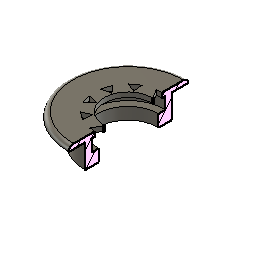
capuchon (Autodesk Fusion 360 design; units mm, degrees)
Autodesk Fusion 360 part; units mm, degrees
sketch "Esquisse1" plane through (0, 0, 0) normal (0, 1, 0) x (1, 0, 0)
  circle A0 centre (0, 0) radius 18.15
  circle A1 centre (0, 0) radius 15.5
  dimension "d1" = 36.3
  dimension "d2" = 31
  constraint coincident A0.centre A1.centre
  constraint concentric A0 A1
  measures "d1" diameter of A0
  measures "d2" diameter of A1
extrude "Extrusion1" add sketch "Esquisse1" along normal blind 10 makes body 1
sketch "Esquisse2" plane through (0, 10, 0) normal (0, 1, 0) x (-1, 0, 0)
  circle A0 centre (0, 0) radius 15.5
  circle A1 centre (0, 0) radius 18.15
  circle A2 centre (0, 0) radius 25
  dimension "d5" = 50
  constraint coincident A0.centre A1.centre
  measures "d5" diameter of A2
extrude "Extrusion2" add sketch "Esquisse2" along normal blind 2 contours A1 | A2 bodies 1
sketch "Esquisse3" plane through (0, 0, 0) normal (0, 1, 0) x (1, 0, 0)
  circle A0 centre (0, 0) radius 16.65
  circle A1 centre (0, 0) radius 12.5
  dimension "d8" = 33.3
  dimension "d9" = 25
  constraint coincident A0.centre A1.centre
  measures "d8" diameter of A0
  measures "d9" diameter of A1
extrude "Extrusion3" add sketch "Esquisse3" along normal blind 5 bodies 1
sketch "Esquisse4" plane through (0, 12, 0) normal (0, 1, 0) x (-1, 0, 0)
  circle A0 centre (0, 0) radius 15.5
  circle A1 centre (0, 0) radius 25
  circle A2 centre (0, 0) radius 16.65
  circle A3 centre (0, 0) radius 10
  dimension "d12" = 33.3
  dimension "d13" = 20
  constraint coincident A0.centre A1.centre
  constraint concentric A2 A3
  measures "d12" diameter of A2
  measures "d13" diameter of A3
extrude "Extrusion4" add sketch "Esquisse4" against normal blind 2 separate body contours A0 makes body 2
fillet "Congé1" radius 2 1 edges at (23.3082, 12, -9.0404) on bodies 1
sketch "Esquisse5" plane through (0, 12, 0) normal (0, 1, 0) x (-1, 0, 0)
  circle A0 centre (0, 0) radius 10
  circle A1 centre (0, 0) radius 15.5
  line L0 (0, 10.5) -> (1.9964, 13.9579)
  line L1 (0, 10.5) -> (3.9928, 10.5) construction
  line L2 (0, 10.5) -> (-2.0557, 13.9579)
  line L3 (-2.0557, 13.9579) -> (1.9964, 13.9579)
  line L4 (-6.1717, 8.4947) -> (-6.5891, 12.4657)
  line L5 (-9.8673, 10.0839) -> (-6.5891, 12.4657)
  line L6 (-6.1717, 8.4947) -> (-9.8673, 10.0839)
  line L7 (-9.9861, 3.2447) -> (-12.6578, 6.2119)
  line L8 (-13.91, 2.3582) -> (-12.6578, 6.2119)
  line L9 (-9.9861, 3.2447) -> (-13.91, 2.3582)
  line L10 (-9.9861, -3.2447) -> (-13.8917, -2.4145)
  line L11 (-12.6395, -6.2683) -> (-13.8917, -2.4145)
  line L12 (-9.9861, -3.2447) -> (-12.6395, -6.2683)
  line L13 (-6.1717, -8.4947) -> (-9.8194, -10.1187)
  line L14 (-6.5412, -12.5005) -> (-9.8194, -10.1187)
  line L15 (-6.1717, -8.4947) -> (-6.5412, -12.5005)
  line L16 (0, -10.5) -> (-1.9964, -13.9579)
  line L17 (2.0557, -13.9579) -> (-1.9964, -13.9579)
  line L18 (0, -10.5) -> (2.0557, -13.9579)
  line L19 (6.1717, -8.4947) -> (6.5891, -12.4657)
  line L20 (9.8673, -10.0839) -> (6.5891, -12.4657)
  line L21 (6.1717, -8.4947) -> (9.8673, -10.0839)
  line L22 (9.9861, -3.2447) -> (12.6578, -6.2119)
  line L23 (13.91, -2.3582) -> (12.6578, -6.2119)
  line L24 (9.9861, -3.2447) -> (13.91, -2.3582)
  line L25 (9.9861, 3.2447) -> (13.8917, 2.4145)
  line L26 (12.6395, 6.2683) -> (13.8917, 2.4145)
  line L27 (9.9861, 3.2447) -> (12.6395, 6.2683)
  line L28 (6.1717, 8.4947) -> (9.8194, 10.1187)
  line L29 (6.5412, 12.5005) -> (9.8194, 10.1187)
  line L30 (6.1717, 8.4947) -> (6.5412, 12.5005)
  dimension "d18" = 60
  dimension "d20" = 360
  constraint horizontal L1
  constraint parallel L1 L3
  measures "d18" angle of L0 L1
extrude "Extrusion5" cut sketch "Esquisse5" against normal blind 5 contours L0 L2 L3 | L4 L5 L6 | L7 L8 L9 | L10 L11 L12 | L13 L14 L15 | L16 L17 L18 | L19 L20 L21 | L22 L23 L24 | L25 L26 L27 | L28 L29 L30 bodies 2
combine "Combiner1" operation add target body 1 tool bodies 2
